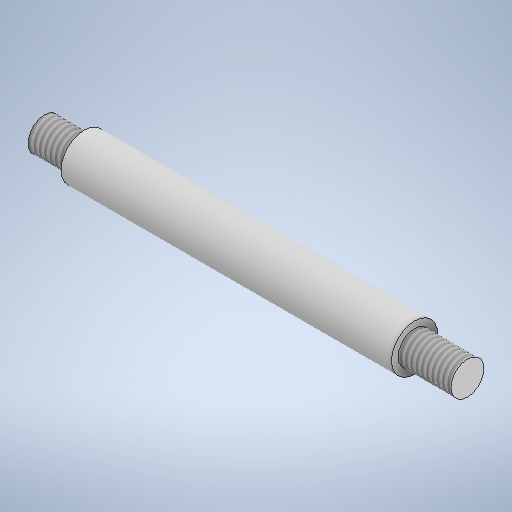
# Autodesk Inventor part: 41
Saved by Autodesk Inventor 2025.1 (Build 291241000, 241)
## iProperties
Created: 2024-09-17
Part Number: 41
Material: Generisch
Document SubType Name: Modeling
Designer: ffogue
Density: 1 g/cm^3
Appearance: Vorgabe
Author: ffogue
Autodesk Inventor part; units mm, degrees
ref_plane "YZ Plane" through (0, 0, 0) normal (1, 0, 0) x (0, 1, 0)
ref_plane "XZ Plane" through (0, 0, 0) normal (0, 1, 0) x (-1, 0, 0)
ref_plane "XY Plane" through (0, 0, 0) normal (0, 0, 1) x (1, 0, 0)
sketch "Sketch1" plane through (0, 0, 0) normal (0, 0, 1) x (1, 0, 0)
  line L0 (0, 0) -> (0, 2.5)
  line L1 (0, 2.5) -> (6, 2.5)
  line L2 (6, 2.5) -> (6, 3.5)
  line L3 (6, 3.5) -> (56, 3.5)
  line L4 (56, 3.5) -> (56, 2.5)
  line L5 (56, 2.5) -> (64, 2.5)
  line L6 (64, 2.5) -> (64, 0)
  line L7 (64, 0) -> (0, 0)
  dimension "d0" = 5
  dimension "d1" = 7
  dimension "d2" = 8
  dimension "d3" = 6
  dimension "d4" = 50
  constraints: 16 end point, 6 perpendicular, 2 point on line, 1 vertical
  measures "d0" diameter of L1 L7
  measures "d1" diameter of L3 L7
  measures "d2" distance of L4.end L5.end
  measures "d3" distance of L0.end L1.end
  measures "d4" distance of L2.end L3.end
revolve "Revolution1" add sketch "Sketch1" angle 360 about axis through (64, 0, 0) along (-1, 0, 0)
thread "Thread1" size "M5x0.8" class "6g" standard "ISO Metric profile" full length
thread "Thread2" size "M5x0.8" class "6g" standard "ISO Metric profile" full length
body "Solid1"
